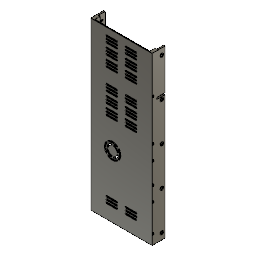
1-CBA_top_Cover_V5 (Autodesk Fusion 360 design; units mm, degrees)
Autodesk Fusion 360 part; units mm, degrees
sketch "Main Profile" plane through (0, 0, 0) normal (0, 0, 1) x (1, 0, 0)
  line L0 (0, 0) -> (-78.5, 0)
  line L1 (-78.5, 0) -> (-78.5, 15)
  line L2 (-78.5, 15) -> (-83.5, 15)
  line L3 (-83.5, 15) -> (-83.5, 35)
  line L4 (-83.5, 35) -> (-88, 35)
  line L5 (-88, 35) -> (-88, -2.8)
  line L6 (-88, -2.8) -> (0, -2.8)
  line L7 (0, -2.8) -> (0, 0)
  line L8 (0, 0) -> (78.5, 0)
  line L9 (88, -2.8) -> (0, -2.8)
  line L10 (78.5, 0) -> (78.5, 15)
  line L11 (78.5, 15) -> (83.5, 15)
  line L12 (83.5, 15) -> (83.5, 35)
  line L13 (83.5, 35) -> (88, 35)
  line L14 (88, 35) -> (88, -2.8)
  dimension "d1" = 78.5
  dimension "d2" = 15
  dimension "d3" = 20
  dimension "d4" = 4.5
  dimension "d5" = 5
  dimension "d6" = 2.8
  constraint coincident L0.start L7.end
  constraint horizontal L0
  constraint perpendicular L0 L1
  constraint perpendicular L1 L2
  constraint perpendicular L0 L3
  constraint perpendicular L3 L4
  constraint perpendicular L0 L5
  constraint perpendicular L3 L6
  constraint vertical L7
  constraint symmetric L0.start L7 L8.start
  constraint symmetric L0.end L7 L8.end
  constraint symmetric L1.end L7 L10.end
  constraint symmetric L2.end L7 L11.end
  constraint symmetric L3.end L7 L12.end
  constraint symmetric L4.end L7 L13.end
  constraint symmetric L5.end L7 L9.start
  constraint symmetric L6.end L7 L9.end
  measures "d1" distance of L0.start L1
  measures "d2" distance of L0 L2
  measures "d3" distance of L2 L4
  measures "d4" distance of L3 L5
  measures "d5" distance of L1 L3
  measures "d6" distance of L0 L6
extrude "Extrude1" add sketch "Main Profile" along normal blind 476.8
sketch "Vents" plane through (0, -2.8, 0) normal (0, -1, 0) x (1, 0, 0)
  line L0 (-88, 0) -> (88, 0)
  line L1 (88, 0) -> (88, 476.8)
  line L2 (88, 476.8) -> (-88, 476.8)
  line L3 (-88, 476.8) -> (-88, 0)
  line L4 (-42, 39.4) -> (-13, 39.4)
  arc A0 (-13, 39.4) -> (-13, 43.4) centre (-13, 41.4) ccw
  line L5 (-13, 43.4) -> (-42, 43.4)
  arc A1 (-42, 43.4) -> (-42, 39.4) centre (-42, 41.4) ccw
  line L6 (-42, 41.4) -> (-13, 41.4) construction
  line L7 (13, 39.4) -> (42, 39.4)
  arc A2 (42, 39.4) -> (42, 43.4) centre (42, 41.4) ccw
  line L8 (42, 43.4) -> (13, 43.4)
  arc A3 (13, 43.4) -> (13, 39.4) centre (13, 41.4) ccw
  line L9 (-42, 47.4) -> (-13, 47.4)
  arc A4 (-13, 47.4) -> (-13, 51.4) centre (-13, 49.4) ccw
  line L10 (-13, 51.4) -> (-42, 51.4)
  arc A5 (-42, 51.4) -> (-42, 47.4) centre (-42, 49.4) ccw
  line L11 (13, 47.4) -> (42, 47.4)
  arc A6 (42, 47.4) -> (42, 51.4) centre (42, 49.4) ccw
  line L12 (42, 51.4) -> (13, 51.4)
  arc A7 (13, 51.4) -> (13, 47.4) centre (13, 49.4) ccw
  line L13 (-42, 55.4) -> (-13, 55.4)
  arc A8 (-13, 55.4) -> (-13, 59.4) centre (-13, 57.4) ccw
  line L14 (-13, 59.4) -> (-42, 59.4)
  arc A9 (-42, 59.4) -> (-42, 55.4) centre (-42, 57.4) ccw
  line L15 (13, 55.4) -> (42, 55.4)
  arc A10 (42, 55.4) -> (42, 59.4) centre (42, 57.4) ccw
  line L16 (42, 59.4) -> (13, 59.4)
  arc A11 (13, 59.4) -> (13, 55.4) centre (13, 57.4) ccw
  arc A12 (-13, 257.4) -> (-13, 261.4) centre (-13, 259.4) ccw
  line L17 (-13, 261.4) -> (-42, 261.4)
  arc A13 (-42, 261.4) -> (-42, 257.4) centre (-42, 259.4) ccw
  line L18 (-42, 257.4) -> (-13, 257.4)
  line L19 (-42, 265.4) -> (-13, 265.4)
  arc A14 (-42, 269.4) -> (-42, 265.4) centre (-42, 267.4) ccw
  line L20 (-13, 269.4) -> (-42, 269.4)
  arc A15 (-13, 265.4) -> (-13, 269.4) centre (-13, 267.4) ccw
  arc A16 (-13, 273.4) -> (-13, 277.4) centre (-13, 275.4) ccw
  line L21 (-13, 277.4) -> (-42, 277.4)
  arc A17 (-42, 277.4) -> (-42, 273.4) centre (-42, 275.4) ccw
  line L22 (-42, 273.4) -> (-13, 273.4)
  line L23 (42, 277.4) -> (13, 277.4)
  arc A18 (42, 273.4) -> (42, 277.4) centre (42, 275.4) ccw
  line L24 (13, 273.4) -> (42, 273.4)
  arc A19 (13, 277.4) -> (13, 273.4) centre (13, 275.4) ccw
  arc A20 (13, 269.4) -> (13, 265.4) centre (13, 267.4) ccw
  line L25 (42, 269.4) -> (13, 269.4)
  line L26 (42, 261.4) -> (13, 261.4)
  line L27 (13, 265.4) -> (42, 265.4)
  arc A21 (42, 265.4) -> (42, 269.4) centre (42, 267.4) ccw
  arc A22 (42, 257.4) -> (42, 261.4) centre (42, 259.4) ccw
  line L28 (13, 257.4) -> (42, 257.4)
  arc A23 (13, 261.4) -> (13, 257.4) centre (13, 259.4) ccw
  line L29 (13, 295.4) -> (42, 295.4)
  line L30 (42, 299.4) -> (13, 299.4)
  line L31 (-42, 295.4) -> (-13, 295.4)
  arc A24 (13, 291.4) -> (13, 287.4) centre (13, 289.4) ccw
  line L32 (13, 303.4) -> (42, 303.4)
  arc A25 (42, 303.4) -> (42, 307.4) centre (42, 305.4) ccw
  arc A26 (-42, 291.4) -> (-42, 287.4) centre (-42, 289.4) ccw
  line L33 (42, 291.4) -> (13, 291.4)
  line L34 (-13, 291.4) -> (-42, 291.4)
  line L35 (13, 287.4) -> (42, 287.4)
  arc A27 (42, 287.4) -> (42, 291.4) centre (42, 289.4) ccw
  arc A28 (-13, 287.4) -> (-13, 291.4) centre (-13, 289.4) ccw
  line L36 (-13, 299.4) -> (-42, 299.4)
  line L37 (42, 307.4) -> (13, 307.4)
  arc A29 (13, 299.4) -> (13, 295.4) centre (13, 297.4) ccw
  arc A30 (13, 307.4) -> (13, 303.4) centre (13, 305.4) ccw
  arc A31 (42, 295.4) -> (42, 299.4) centre (42, 297.4) ccw
  arc A32 (-13, 303.4) -> (-13, 307.4) centre (-13, 305.4) ccw
  arc A33 (-42, 299.4) -> (-42, 295.4) centre (-42, 297.4) ccw
  line L38 (-42, 287.4) -> (-13, 287.4)
  line L39 (-13, 307.4) -> (-42, 307.4)
  arc A34 (-13, 295.4) -> (-13, 299.4) centre (-13, 297.4) ccw
  line L40 (-42, 303.4) -> (-13, 303.4)
  arc A35 (-42, 307.4) -> (-42, 303.4) centre (-42, 305.4) ccw
  line L41 (13, 325.4) -> (42, 325.4)
  line L42 (42, 329.4) -> (13, 329.4)
  line L43 (-42, 325.4) -> (-13, 325.4)
  arc A36 (13, 321.4) -> (13, 317.4) centre (13, 319.4) ccw
  line L44 (13, 333.4) -> (42, 333.4)
  arc A37 (42, 333.4) -> (42, 337.4) centre (42, 335.4) ccw
  arc A38 (-42, 321.4) -> (-42, 317.4) centre (-42, 319.4) ccw
  line L45 (42, 321.4) -> (13, 321.4)
  line L46 (-13, 321.4) -> (-42, 321.4)
  line L47 (13, 317.4) -> (42, 317.4)
  arc A39 (42, 317.4) -> (42, 321.4) centre (42, 319.4) ccw
  arc A40 (-13, 317.4) -> (-13, 321.4) centre (-13, 319.4) ccw
  line L48 (-13, 329.4) -> (-42, 329.4)
  line L49 (42, 337.4) -> (13, 337.4)
  arc A41 (13, 329.4) -> (13, 325.4) centre (13, 327.4) ccw
  arc A42 (13, 337.4) -> (13, 333.4) centre (13, 335.4) ccw
  arc A43 (42, 325.4) -> (42, 329.4) centre (42, 327.4) ccw
  arc A44 (-13, 333.4) -> (-13, 337.4) centre (-13, 335.4) ccw
  arc A45 (-42, 329.4) -> (-42, 325.4) centre (-42, 327.4) ccw
  line L50 (-42, 317.4) -> (-13, 317.4)
  line L51 (-13, 337.4) -> (-42, 337.4)
  arc A46 (-13, 325.4) -> (-13, 329.4) centre (-13, 327.4) ccw
  line L52 (-42, 333.4) -> (-13, 333.4)
  arc A47 (-42, 337.4) -> (-42, 333.4) centre (-42, 335.4) ccw
  line L53 (13, 385.4) -> (42, 385.4)
  line L54 (42, 389.4) -> (13, 389.4)
  line L55 (-42, 385.4) -> (-13, 385.4)
  arc A48 (13, 381.4) -> (13, 377.4) centre (13, 379.4) ccw
  line L56 (13, 393.4) -> (42, 393.4)
  arc A49 (42, 393.4) -> (42, 397.4) centre (42, 395.4) ccw
  arc A50 (-42, 381.4) -> (-42, 377.4) centre (-42, 379.4) ccw
  line L57 (42, 381.4) -> (13, 381.4)
  line L58 (-13, 381.4) -> (-42, 381.4)
  line L59 (13, 377.4) -> (42, 377.4)
  arc A51 (42, 377.4) -> (42, 381.4) centre (42, 379.4) ccw
  arc A52 (-13, 377.4) -> (-13, 381.4) centre (-13, 379.4) ccw
  line L60 (-13, 389.4) -> (-42, 389.4)
  line L61 (42, 397.4) -> (13, 397.4)
  arc A53 (13, 389.4) -> (13, 385.4) centre (13, 387.4) ccw
  arc A54 (13, 397.4) -> (13, 393.4) centre (13, 395.4) ccw
  arc A55 (42, 385.4) -> (42, 389.4) centre (42, 387.4) ccw
  arc A56 (-13, 393.4) -> (-13, 397.4) centre (-13, 395.4) ccw
  arc A57 (-42, 389.4) -> (-42, 385.4) centre (-42, 387.4) ccw
  line L62 (-42, 377.4) -> (-13, 377.4)
  line L63 (-13, 397.4) -> (-42, 397.4)
  arc A58 (-13, 385.4) -> (-13, 389.4) centre (-13, 387.4) ccw
  line L64 (-42, 393.4) -> (-13, 393.4)
  arc A59 (-42, 397.4) -> (-42, 393.4) centre (-42, 395.4) ccw
  line L65 (13, 415.4) -> (42, 415.4)
  line L66 (42, 419.4) -> (13, 419.4)
  line L67 (-42, 415.4) -> (-13, 415.4)
  arc A60 (13, 411.4) -> (13, 407.4) centre (13, 409.4) ccw
  line L68 (13, 423.4) -> (42, 423.4)
  arc A61 (42, 423.4) -> (42, 427.4) centre (42, 425.4) ccw
  arc A62 (-42, 411.4) -> (-42, 407.4) centre (-42, 409.4) ccw
  line L69 (42, 411.4) -> (13, 411.4)
  line L70 (-13, 411.4) -> (-42, 411.4)
  line L71 (13, 407.4) -> (42, 407.4)
  arc A63 (42, 407.4) -> (42, 411.4) centre (42, 409.4) ccw
  arc A64 (-13, 407.4) -> (-13, 411.4) centre (-13, 409.4) ccw
  line L72 (-13, 419.4) -> (-42, 419.4)
  line L73 (42, 427.4) -> (13, 427.4)
  arc A65 (13, 419.4) -> (13, 415.4) centre (13, 417.4) ccw
  arc A66 (13, 427.4) -> (13, 423.4) centre (13, 425.4) ccw
  arc A67 (42, 415.4) -> (42, 419.4) centre (42, 417.4) ccw
  arc A68 (-13, 423.4) -> (-13, 427.4) centre (-13, 425.4) ccw
  arc A69 (-42, 419.4) -> (-42, 415.4) centre (-42, 417.4) ccw
  line L74 (-42, 407.4) -> (-13, 407.4)
  line L75 (-13, 427.4) -> (-42, 427.4)
  arc A70 (-13, 415.4) -> (-13, 419.4) centre (-13, 417.4) ccw
  line L76 (-42, 423.4) -> (-13, 423.4)
  arc A71 (-42, 427.4) -> (-42, 423.4) centre (-42, 425.4) ccw
  line L77 (13, 445.4) -> (42, 445.4)
  line L78 (42, 449.4) -> (13, 449.4)
  line L79 (-42, 445.4) -> (-13, 445.4)
  arc A72 (13, 441.4) -> (13, 437.4) centre (13, 439.4) ccw
  line L80 (13, 453.4) -> (42, 453.4)
  arc A73 (42, 453.4) -> (42, 457.4) centre (42, 455.4) ccw
  arc A74 (-42, 441.4) -> (-42, 437.4) centre (-42, 439.4) ccw
  line L81 (42, 441.4) -> (13, 441.4)
  line L82 (-13, 441.4) -> (-42, 441.4)
  line L83 (13, 437.4) -> (42, 437.4)
  arc A75 (42, 437.4) -> (42, 441.4) centre (42, 439.4) ccw
  arc A76 (-13, 437.4) -> (-13, 441.4) centre (-13, 439.4) ccw
  line L84 (-13, 449.4) -> (-42, 449.4)
  line L85 (42, 457.4) -> (13, 457.4)
  arc A77 (13, 449.4) -> (13, 445.4) centre (13, 447.4) ccw
  arc A78 (13, 457.4) -> (13, 453.4) centre (13, 455.4) ccw
  arc A79 (42, 445.4) -> (42, 449.4) centre (42, 447.4) ccw
  arc A80 (-13, 453.4) -> (-13, 457.4) centre (-13, 455.4) ccw
  arc A81 (-42, 449.4) -> (-42, 445.4) centre (-42, 447.4) ccw
  line L86 (-42, 437.4) -> (-13, 437.4)
  line L87 (-13, 457.4) -> (-42, 457.4)
  arc A82 (-13, 445.4) -> (-13, 449.4) centre (-13, 447.4) ccw
  line L88 (-42, 453.4) -> (-13, 453.4)
  arc A83 (-42, 457.4) -> (-42, 453.4) centre (-42, 455.4) ccw
  arc A84 (-29.1219, 194.5801) -> (-41.1246, 182.4441) centre (-25, 178.5) ccw
  arc A85 (-28.2776, 191.2866) -> (-29.1219, 194.5801) centre (-28.6998, 192.9334) ccw
  arc A86 (-28.2776, 191.2866) -> (-37.822, 181.6363) centre (-25, 178.5) ccw
  arc A87 (-41.1246, 182.4441) -> (-37.822, 181.6363) centre (-39.4733, 182.0402) ccw
  arc A88 (-28.6998, 192.9334) -> (-39.4733, 182.0402) centre (-25, 178.5) ccw construction
  arc A89 (-41.3077, 189.9048) -> (-41.2401, 166.9992) centre (-25, 178.5) ccw
  arc A90 (-41.3077, 189.9048) -> (-44.0939, 191.8533) centre (-42.7008, 190.8791) ccw
  arc A91 (-44.0939, 191.8533) -> (-44.0148, 165.0343) centre (-25, 178.5) ccw
  arc A92 (-44.0148, 165.0343) -> (-41.2401, 166.9992) centre (-42.6275, 166.0167) ccw
  arc A93 (-42.7008, 190.8791) -> (-42.6275, 166.0167) centre (-25, 178.5) ccw construction
  line L89 (-25, 178.5) -> (-29.91, 178.5) construction
  arc A94 (-36.4048, 162.1923) -> (-38.3533, 159.4061) centre (-37.3791, 160.7992) ccw
  arc A95 (-36.4048, 162.1923) -> (-13.4992, 162.2599) centre (-25, 178.5) ccw
  arc A96 (-38.3533, 159.4061) -> (-11.5343, 159.4852) centre (-25, 178.5) ccw
  arc A97 (-11.5343, 159.4852) -> (-13.4992, 162.2599) centre (-12.5167, 160.8725) ccw
  arc A98 (-37.7866, 175.2224) -> (-28.1363, 165.678) centre (-25, 178.5) ccw
  arc A99 (-41.0801, 174.3781) -> (-28.9441, 162.3754) centre (-25, 178.5) ccw
  arc A100 (-37.7866, 175.2224) -> (-41.0801, 174.3781) centre (-39.4334, 174.8002) ccw
  arc A101 (-28.9441, 162.3754) -> (-28.1363, 165.678) centre (-28.5402, 164.0267) ccw
  arc A102 (-8.6923, 167.0952) -> (-5.9061, 165.1467) centre (-7.2992, 166.1209) ccw
  arc A103 (-8.6923, 167.0952) -> (-8.7599, 190.0008) centre (-25, 178.5) ccw
  arc A104 (-5.9061, 165.1467) -> (-5.9852, 191.9657) centre (-25, 178.5) ccw
  arc A105 (-5.9852, 191.9657) -> (-8.7599, 190.0008) centre (-7.3725, 190.9833) ccw
  arc A106 (-21.7224, 165.7134) -> (-12.178, 175.3637) centre (-25, 178.5) ccw
  arc A107 (-20.8781, 162.4199) -> (-8.8754, 174.5559) centre (-25, 178.5) ccw
  arc A108 (-21.7224, 165.7134) -> (-20.8781, 162.4199) centre (-21.3002, 164.0666) ccw
  arc A109 (-8.8754, 174.5559) -> (-12.178, 175.3637) centre (-10.5267, 174.9598) ccw
  arc A110 (-13.5952, 194.8077) -> (-11.6467, 197.5939) centre (-12.6209, 196.2008) ccw
  arc A111 (-13.5952, 194.8077) -> (-36.5008, 194.7401) centre (-25, 178.5) ccw
  arc A112 (-11.6467, 197.5939) -> (-38.4657, 197.5148) centre (-25, 178.5) ccw
  arc A113 (-38.4657, 197.5148) -> (-36.5008, 194.7401) centre (-37.4833, 196.1275) ccw
  arc A114 (-12.2134, 181.7776) -> (-21.8637, 191.322) centre (-25, 178.5) ccw
  arc A115 (-8.9199, 182.6219) -> (-21.0559, 194.6246) centre (-25, 178.5) ccw
  arc A116 (-12.2134, 181.7776) -> (-8.9199, 182.6219) centre (-10.5666, 182.1998) ccw
  arc A117 (-21.0559, 194.6246) -> (-21.8637, 191.322) centre (-21.4598, 192.9733) ccw
  dimension "d9" = 4
  dimension "d10" = 41.4
  dimension "d11" = 13
  dimension "d12" = 29
  dimension "d15" = 55
  dimension "d16" = 8
  dimension "d19" = 0
  dimension "d20" = 218
  dimension "d23" = 0
  dimension "d24" = 30
  dimension "d26" = 178.5
  dimension "d27" = 25
  dimension "d28" = 14.9
  dimension "d29" = 3.4
  dimension "d30" = 3.4
  dimension "d31" = 21.6
  dimension "d32" = 75.623
  dimension "d33" = 13.745
  dimension "d35" = 35.305
  dimension "d36" = 44.063
  dimension "d38" = 360
  constraint tangent L4 A0
  constraint tangent A0 L5
  constraint parallel L4 L5
  constraint tangent L5 A1
  constraint tangent L4 A1
  constraint horizontal L6
  constraint tangent A84 A85
  constraint tangent A85 A86
  constraint tangent A86 A87
  constraint tangent A84 A87
  constraint tangent A89 A90
  constraint tangent A90 A91
  constraint tangent A91 A92
  constraint tangent A89 A92
  constraint coincident A84.centre A86.centre
  constraint horizontal L89
  measures "d9" diameter of A0
  measures "d10" distance of origin L6
  measures "d11" horizontal distance of origin A0.centre
  measures "d12" distance of A1.centre A0.centre
  measures "d26" distance of L0 A84.centre
  measures "d27" horizontal distance of origin A84.centre
  measures "d28" radius of A88
  measures "d29" distance of A84 A86
  measures "d30" distance of A89 A91
  measures "d31" radius of A93
  measures "d32" angle of A85.centre A84.centre L89.end
  measures "d33" angle of A87.centre A84.centre L89.end
  measures "d35" angle of A92.centre A84.centre L89.end
  measures "d36" angle of A84.centre A90.centre L89.end
extrude "Extrude2" cut sketch "Vents" against normal blind 20 contours L4 A0 L5 A1 | L7 A2 L8 A3 | L9 A4 L10 A5 | L11 A6 L12 A7 | L13 A8 L14 A9 | L15 A10 L16 A11 | A12 L17 A13 L18 | L19 A14 L20 A15 | A16 L21 A17 L22 | L23 A18 L24 A19 | A20 L25 L27 A21 | L26 A22 L28 A23 | L29 L30 A29 A31 | L31 L36 A33 A34 | A24 L33 L35 A27 | L32 A25 L37 A30 | A26 L34 A28 L38 | A32 L39 L40 A35 | L41 L42 A41 A43 | L43 L48 A45 A46 | A36 L45 L47 A39 | L44 A37 L49 A42 | A38 L46 A40 L50 | A44 L51 L52 A47 | L53 L54 A53 A55 | L55 L60 A57 A58 | A48 L57 L59 A51 | L56 A49 L61 A54 | A50 L58 A52 L62 | A56 L63 L64 A59 | L65 L66 A65 A67 | L67 L72 A69 A70 | A60 L69 L71 A63 | L68 A61 L73 A66 | A62 L70 A64 L74 | A68 L75 L76 A71 | L77 L78 A77 A79 | L79 L84 A81 A82 | A72 L81 L83 A75 | L80 A73 L85 A78 | A74 L82 A76 L86 | A80 L87 L88 A83 | A84 A85 A86 A87 | A89 A90 A91 A92 | A94 A95 A96 A97 | A98 A99 A100 A101 | A102 A103 A104 A105 | A106 A107 A108 A109 | A110 A111 A112 A113 | A114 A115 A116 A117
sketch "Side" plane through (88, 0, 0) normal (1, 0, 0) x (0, 1, 0)
  line L0 (-2.8, 0) -> (35, 0)
  line L1 (35, 0) -> (35, 476.8)
  line L2 (35, 476.8) -> (-2.8, 476.8)
  line L3 (-2.8, 476.8) -> (-2.8, 0)
  circle A0 centre (25, 18.5) radius 2.75
  circle A1 centre (25, 18.5) radius 5
  circle A2 centre (25, 128.5) radius 2.75
  circle A3 centre (25, 128.5) radius 5
  circle A4 centre (25, 238.5) radius 2.75
  circle A5 centre (25, 238.5) radius 5
  circle A6 centre (25, 348.5) radius 2.75
  circle A7 centre (25, 348.5) radius 5
  circle A8 centre (25, 458.5) radius 2.75
  circle A9 centre (25, 458.5) radius 5
  line L4 (0, 24.5) -> (2, 24.5)
  line L5 (2, 24.5) -> (2, 30.5)
  line L6 (2, 30.5) -> (0, 30.5)
  line L7 (0, 30.5) -> (0, 24.5)
  line L8 (0, 0) -> (0, 476.8)
  line L9 (2, 109.4) -> (0, 109.4)
  line L10 (0, 109.4) -> (0, 103.4)
  line L11 (0, 103.4) -> (2, 103.4)
  line L12 (2, 103.4) -> (2, 109.4)
  line L13 (2, 151.4) -> (0, 151.4)
  line L14 (0, 151.4) -> (0, 145.4)
  line L15 (0, 145.4) -> (2, 145.4)
  line L16 (2, 145.4) -> (2, 151.4)
  line L17 (0, 253.4) -> (0, 247.4)
  line L18 (0, 211.4) -> (0, 205.4)
  line L19 (0, 205.4) -> (2, 205.4)
  line L20 (2, 205.4) -> (2, 211.4)
  line L21 (2, 211.4) -> (0, 211.4)
  line L22 (0, 247.4) -> (2, 247.4)
  line L23 (2, 247.4) -> (2, 253.4)
  line L24 (2, 253.4) -> (0, 253.4)
  line L25 (0, 371.4) -> (0, 365.4)
  line L26 (2, 371.4) -> (0, 371.4)
  line L27 (2, 365.4) -> (2, 371.4)
  line L28 (0, 365.4) -> (2, 365.4)
  line L29 (12.4, 216) -> (43.0626, 216)
  arc A10 (43.0626, 216) -> (43.0626, 221) centre (43.0626, 218.5) ccw
  line L30 (43.0626, 221) -> (12.4, 221)
  arc A11 (12.4, 221) -> (12.4, 216) centre (12.4, 218.5) ccw
  line L31 (12.4, 218.5) -> (43.0626, 218.5) construction
  line L32 (43.0626, 360.9) -> (12.4, 360.9)
  arc A12 (12.4, 360.9) -> (12.4, 355.9) centre (12.4, 358.4) ccw
  line L33 (12.4, 355.9) -> (43.0626, 355.9)
  arc A13 (43.0626, 355.9) -> (43.0626, 360.9) centre (43.0626, 358.4) ccw
  dimension "d41" = 5.5
  dimension "d42" = 10
  dimension "d43" = 10
  dimension "d44" = 18.5
  dimension "d47" = 0
  dimension "d48" = 110
  dimension "d49" = 6
  dimension "d50" = 2
  dimension "d51" = 24.5
  dimension "d54" = 0
  dimension "d55" = 78.9
  dimension "d58" = 0
  dimension "d59" = 42
  dimension "d62" = 0
  dimension "d63" = 102
  dimension "d66" = 0
  dimension "d67" = 118
  dimension "d68" = 5
  dimension "d69" = 22.6
  dimension "d70" = 218.5
  dimension "d73" = 0
  dimension "d74" = 139.9
  constraint concentric A0 A1
  constraint horizontal L4
  constraint vertical L5
  constraint horizontal L6
  constraint vertical L7
  constraint coincident L4.start L8
  constraint tangent L29 A10
  constraint tangent A10 L30
  constraint parallel L29 L30
  constraint tangent L30 A11
  constraint tangent L29 A11
  constraint horizontal L31
  measures "d41" diameter of A0
  measures "d42" diameter of A1
  measures "d43" distance of L1 A0.centre
  measures "d44" distance of L0 A0.centre
  measures "d49" distance of L4 L6
  measures "d50" distance of L5 L7
  measures "d51" distance of L0 L4
  measures "d68" diameter of A10
  measures "d69" distance of L1 A11.centre
  measures "d70" distance of L0 L31
extrude "Extrude3" cut sketch "Side" against normal blind 27.382 contours L1 L32 L33 A13 | L1 L32 A12 L33
extrude "Extrude4" cut sketch "Side" along normal blind 20 from surface at -176 contours L1 L29 L30 A11 | L1 L29 A10 L30
extrude "Extrude5" cut sketch "Side" against normal blind 350 contours L4 L5 L6 L7 L8 | L8 L25 L26 L27 L28 | L8 L9 L10 L11 L12 | L8 L17 L22 L23 L24 | L8 L13 L14 L15 L16 | L8 L18 L19 L20 L21
extrude "Extrude6" cut sketch "Side" against normal blind 10 contours A0 | A2 | A4 | A6 | A8
extrude "Extrude7" cut sketch "Side" against normal blind 1.5 contours A1 | A3 | A5 | A7 | A9
mirror "Mirror1" about plane through (0, 0, 0) normal (1, 0, 0) of "Extrude6", "Extrude7"
named bodies: "1-CBA top Cover V5"
